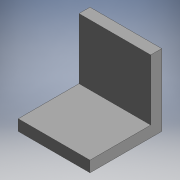
# Autodesk Inventor part: Part16
Saved by Autodesk Inventor 2016 (Build 200138000, 138)
## iProperties
Created: 2018-01-18
Part Number: Part16
Material: Generic
Document SubType Name: Modeling
Designer: student
Density: 1 g/cm^3
Appearance: Default
Author: student
Autodesk Inventor part; units mm, degrees
ref_plane "YZ Plane" through (0, 0, 0) normal (1, 0, 0) x (0, 1, 0)
ref_plane "XZ Plane" through (0, 0, 0) normal (0, 1, 0) x (-1, 0, 0)
ref_plane "XY Plane" through (0, 0, 0) normal (0, 0, 1) x (1, 0, 0)
sketch "Sketch1" plane through (0, 0, 0) normal (0, 1, 0) x (-1, 0, 0)
  line L0 (-13.4529, -30.7592) -> (5.5971, -30.7592)
  line L1 (5.5971, -30.7592) -> (5.5971, -49.8092)
  line L2 (5.5971, -49.8092) -> (-13.4529, -49.8092)
  line L3 (-13.4529, -49.8092) -> (-13.4529, -30.7592)
  line L4 (-13.4529, -30.7592) -> (5.5971, -49.8092) construction
  line L5 (5.5971, -30.7592) -> (-13.4529, -49.8092) construction
  point P0 (0, 0)
  point P1 (-3.9279, -40.2842)
  dimension "d0" = 19.05
  dimension "d1" = 19.05
  constraints: 12 end point, 2 midpoint, 2 parallel, 1 horizontal, 1 perpendicular
  measures "d0" distance of L1.end L2.end
  measures "d1" distance of L0.end L1.end
extrude "Extrusion1" add sketch "Sketch1" along normal blind 2.921
sketch "Sketch2" plane through (0, 2.921, 0) normal (0, 1, 0) x (1, 0, 0)
  line L0 (-5.5971, 49.8092) -> (13.4529, 49.8092)
  line L1 (13.4529, 49.8092) -> (13.4529, 46.8882)
  line L2 (13.4529, 46.8882) -> (-5.5971, 46.8882)
  line L3 (-5.5971, 46.8882) -> (-5.5971, 49.8092)
  point P0 (0, 0)
  dimension "d4" = 19.05
  dimension "d5" = 2.921
  constraints: 8 end point, 2 parallel, 1 horizontal, 1 perpendicular
  measures "d4" distance of L1.end L2.end
  measures "d5" distance of L0.end L1.end
extrude "Extrusion2" add sketch "Sketch2" along normal blind 16.129
body "Solid1"
